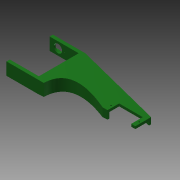
# Autodesk Inventor part: arm2
Saved by Autodesk Inventor 2013 (Build 170138000, 138)
## iProperties
Created: 2014-06-28
Part Number: arm2
Material: Generic
Document SubType Name: Modeling
Designer: Masta
Density: 1 g/cm^3
Author: Masta
Autodesk Inventor part; units mm, degrees
note: some values were not read from the file. Chosen so that the rebuilt part matches the saved one: direction of "Hole1".
ref_plane "YZ Plane" through (0, 0, 0) normal (1, 0, 0) x (0, 1, 0)
ref_plane "XZ Plane" through (0, 0, 0) normal (0, 1, 0) x (-1, 0, 0)
ref_plane "XY Plane" through (0, 0, 0) normal (0, 0, 1) x (1, 0, 0)
sketch "Sketch1" plane through (0, 0, 0) normal (0, 0, 1) x (1, 0, 0)
  line L0 (0, 0) -> (35, 0)
  line L1 (35, 0) -> (35, 48)
  line L2 (35, 48) -> (0, 48)
  line L3 (0, 48) -> (0, 0) construction
  line L4 (0, 48) -> (0, 50)
  line L5 (0, 50) -> (39, 50)
  line L6 (39, 50) -> (39, -4)
  line L7 (39, -4) -> (0, -4)
  line L8 (0, -4) -> (0, 0)
  line L9 (10, 0) -> (10, 48) construction
  dimension "d0" = 35
  dimension "d1" = 48
  dimension "d2" = 2
  dimension "d3" = 4
  dimension "d4" = 4
  dimension "d30" = 10
  constraints: 20 end point, 4 perpendicular, 3 parallel, 2 collinear, 2 point on line, 1 horizontal
  measures "d0" distance of L0.start L0.end
  measures "d1" distance of L0.end L1.end
  measures "d2" distance of L2.end L4.end
  measures "d3" distance of L7.end L0.start
  measures "d4" distance between parallel lines of L1 L6
  measures "d30" distance between parallel lines of L9 L3
extrude "Extrusion1" add sketch "Sketch1" along normal mid plane 15
sketch "Sketch2" plane through (0, 0, 7.5) normal (0, 1, 0) x (1, 0, 0)
  line L0 (0, 15) -> (35, 15) projected
  line L1 (0, 7.5) -> (10, 7.5) construction
  circle A0 centre (10, 7.5) radius 2.5
  circle A1 centre (10, 7.5) radius 3.5
  dimension "d7" = 10
  dimension "d8" = 5
  dimension "d9" = 7
  constraints: 2 centre point, 2 coincident, 2 end point, 1 parallel
  measures "d7" distance of L1.start L1.end
  measures "d8" diameter of A0
  measures "d9" diameter of A1
extrude "Extrusion2" add sketch "Sketch2" along normal blind 1 contours A0 | A1
extrude "Extrusion3" add sketch "Sketch2" along normal blind 4 draft -10 contours A0
fillet "Fillet1" radius 2 1 edges at (8.2053, 4, 0)
sketch "Sketch3" plane through (0, 50, 7.5) normal (0, 1, 0) x (1, 0, 0)
  line L0 (39, 0) -> (39, 15) projected
  line L1 (0, 15) -> (39, 15) projected
  line L2 (39, 15) -> (39, 0) projected
  line L3 (39, 0) -> (0, 0) projected
  line L4 (0, 0) -> (0, 15) projected
  circle A0 centre (10, 7.5) radius 3.5 construction
  circle A1 centre (10, 7.5) radius 5
  line L5 (39, 12) -> (0, 12)
  line L6 (0, 12) -> (0, 3)
  line L7 (0, 3) -> (39, 3)
  line L8 (39, 3) -> (39, 12)
  line L9 (39, 12) -> (0, 3) construction
  line L10 (0, 12) -> (39, 3) construction
  line L11 (10, 7.5) -> (19.5, 7.5) construction
  line L12 (10, 7.5) -> (17.62, 7.5) construction
  line L13 (17.62, 7.5) -> (29.62, 7.5) construction
  point P0 (0, 7.5)
  dimension "d15" = 10
  dimension "d16" = 9
  dimension "d21" = 7.62
  dimension "d22" = 12
  constraints: 18 end point, 3 coincident, 2 collinear, 2 midpoint, 2 parallel, 2 perpendicular, 2 point on line, 1 centre point, 1 horizontal
  measures "d15" diameter of A1
  measures "d16" distance of L5.end L6.end
  measures "d21" distance of L11.start L12.end
  measures "d22" distance of L12.end L13.end
extrude "Extrusion4" cut sketch "Sketch3" against normal up to next contours L7 A1 L5 | A1 L7 | L5 A1
extrude "Extrusion5" add sketch "Sketch3" along normal blind 2 contours L3 L4 L7 A1 L0 | L5 A1 L4 L1 L0
hole "Hole1" at (17.62, 50, 0) at (29.62, 50, 0) direction (0, -1, 0) diameter 1 end up to surface
sketch "Sketch4" plane through (0, 0, 7.5) normal (0, 0, 1) x (1, 0, 0)
  line L0 (0, -4) -> (39, -4) projected
  line L1 (39, -4) -> (39, 52) projected
  line L2 (35, 48) -> (35, 0) projected
  line L3 (39, 13) -> (126, 13) construction
  line L4 (10, 0) -> (10, 48) construction
  line L5 (140.25, 6) -> (111.75, 6) construction
  line L6 (111.75, 6) -> (111.75, 20)
  line L7 (111.75, 20) -> (140.25, 20)
  line L8 (140.25, 20) -> (140.25, 6)
  line L9 (140.25, 6) -> (111.75, 20) construction
  line L10 (111.75, 6) -> (140.25, 20) construction
  line L11 (140.25, 6) -> (145.25, 6)
  line L12 (145.25, 6) -> (145.25, 25)
  line L13 (145.25, 25) -> (39, 52)
  line L14 (39, 49.4205) -> (145.25, 22.4205)
  line L15 (126, 13) -> (145.25, 13) construction
  line L16 (111.75, 6) -> (105.75, 6)
  spline S0 degree 2 poles (45, -4) (45.7494, 31.9198) (105.75, 6) knots 0 0 0 1 1 1
  line L17 (45, -4) -> (39, -4)
  line L18 (111.75, 8) -> (106.1627, 8)
  line L19 (43.0862, -2) -> (39, -2)
  spline S1 degree 5 poles (106.1627, 8) (102.5942, 9.5347) (98.9966, 11.0018) (95.3666, 12.3881) (88.7121, 14.7258) (81.921, 16.6254) (78.8427, 17.3692) (73.2935, 18.4553) (67.6605, 18.92) (65.1757, 18.9754) (60.6409, 18.722) (56.2516, 17.5949) (54.3261, 16.8749) (50.7846, 14.9574) (47.9251, 12.1267) (46.7443, 10.5387) (44.892, 7.1897) (43.8107, 3.5191) (43.4465, 1.6935) (43.2118, -0.1496) (43.0862, -2) knots 0 0 0 0 0 0 0.252764 0.252764 0.252764 0.458659 0.458659 0.458659 0.620049 0.620049 0.620049 0.752463 0.752463 0.752463 0.879316 0.879316 0.879316 1 1 1 1 1 1
  point P0 (143, 13)
  point P1 (109, 13)
  point P2 (54.4891, 14.558)
  dimension "d39" = 116
  dimension "d40" = 28.5
  dimension "d41" = 14
  dimension "d42" = 5
  dimension "d43" = 5
  dimension "d44" = 2.5
  dimension "d45" = 10
  dimension "d46" = 17
  dimension "d47" = 17
  dimension "d48" = 6
  dimension "d49" = 6
  dimension "d50" = 2
  constraints: 32 end point, 8 parallel, 8 point on line, 5 perpendicular, 2 midpoint, 1 horizontal, 6 other
  measures "d39" distance from line of L3.end L4
  measures "d40" distance of L6.end L7.end
  measures "d41" distance of L5.end L6.end
  measures "d42" distance of L5.start L11.end
  measures "d43" distance from line of L12.end L7
  measures "d44" distance between parallel lines of L13 L14
  measures "d45" distance between parallel lines of L0 L5
  measures "d46" distance of L3.end point (109, 13)
  measures "d47" distance of point (143, 13) L3.end
  measures "d48" distance of L5.end L16.end
  measures "d49" distance of L17.start L0.end
  measures "d50" distance between parallel lines of L16 L18
extrude "Extrusion6" add sketch "Sketch4" against normal blind 3
extrude "Extrusion7" add sketch "Sketch4" against normal up to surface (15 mm away) contours L1 L19 S1 L18 L6 L16 S0 L17 | L1 L13 L12 L14
sketch "Sketch5" plane through (0, 52, 7.5) normal (0, 1, 0) x (1, 0, 0)
  line L0 (145.25, 0) -> (39, 0) projected
  line L1 (145.25, 0) -> (145.25, 15) projected
  line L2 (39, 15) -> (145.25, 15) projected
  line L3 (39, 12) -> (39, 15) projected
  line L4 (39, 3) -> (39, 12) projected
  line L5 (39, 0) -> (39, 3) projected
  line L6 (39, 15) -> (145.25, 7.5)
  line L7 (145.25, 7.5) -> (145.25, 15)
  line L8 (39, 15) -> (145.25, 15)
  point P0 (0, 7.5)
  constraints: 6 end point, 2 collinear, 1 midpoint
extrude "Extrusion8" cut sketch "Sketch5" against normal through all contours L6 L2 L1
hole "Hole2" at (143, 13, 7.5) at (109, 13, 7.5) direction (0, 0, -1) diameter 1.5 end through all
body "Solid1"
